Autodesk Inventor part; units mm, degrees
(part 2 of 3)
sketch "Sketch3" plane through (0, 0, 0) normal (0, 0, -1) x (-1, 0, 0)
  line L0 (-53.5235, -6.5875) -> (-53.5235, 0.9125)
  line L1 (5.4544, -6.5875) -> (-53.5235, -6.5875)
  line L2 (5.4544, 0.9125) -> (5.4544, -6.5875)
  line L3 (2.5944, 0.9125) -> (5.4544, 0.9125)
  arc A0 (2.5944, 0.9125) -> (2.4065, 0.7809) centre (2.5944, 0.7125) ccw
  line L4 (2.2868, 0.452) -> (2.4065, 0.7809)
  arc A1 (2.0617, 0.2877) -> (2.2868, 0.452) centre (2.0518, 0.5375) ccw
  arc A2 (2.0617, 0.2877) -> (2.0715, 0.2875) centre (2.0715, 0.5375) ccw
  line L5 (2.0518, 0.2875) -> (2.0715, 0.2875)
  arc A3 (2.0518, 0.2875) -> (2.0617, 0.2877) centre (2.0518, 0.5375) ccw
  arc A4 (1.8366, 0.452) -> (2.0617, 0.2877) centre (2.0715, 0.5375) ccw
  line L6 (1.5109, 1.3467) -> (1.8366, 0.452)
  arc A5 (1.5109, 1.3467) -> (1.417, 1.4125) centre (1.417, 1.3125) ccw
  line L7 (1.1356, 1.4125) -> (1.417, 1.4125)
  arc A6 (1.1356, 1.4125) -> (1.0416, 1.3467) centre (1.1356, 1.3125) ccw
  line L8 (0.716, 0.452) -> (1.0416, 1.3467)
  arc A7 (0.4909, 0.2877) -> (0.716, 0.452) centre (0.481, 0.5375) ccw
  arc A8 (0.4909, 0.2877) -> (0.5007, 0.2875) centre (0.5007, 0.5375) ccw
  line L9 (0.481, 0.2875) -> (0.5007, 0.2875)
  arc A9 (0.481, 0.2875) -> (0.4909, 0.2877) centre (0.481, 0.5375) ccw
  arc A10 (0.2658, 0.452) -> (0.4909, 0.2877) centre (0.5007, 0.5375) ccw
  line L10 (-0.0599, 1.3467) -> (0.2658, 0.452)
  arc A11 (-0.0599, 1.3467) -> (-0.1538, 1.4125) centre (-0.1538, 1.3125) ccw
  line L11 (-0.4352, 1.4125) -> (-0.1538, 1.4125)
  arc A12 (-0.4352, 1.4125) -> (-0.5292, 1.3467) centre (-0.4352, 1.3125) ccw
  line L12 (-0.8548, 0.452) -> (-0.5292, 1.3467)
  arc A13 (-1.0799, 0.2877) -> (-0.8548, 0.452) centre (-1.0898, 0.5375) ccw
  arc A14 (-1.0799, 0.2877) -> (-1.0701, 0.2875) centre (-1.0701, 0.5375) ccw
  line L13 (-1.0898, 0.2875) -> (-1.0701, 0.2875)
  arc A15 (-1.0898, 0.2875) -> (-1.0799, 0.2877) centre (-1.0898, 0.5375) ccw
  arc A16 (-1.305, 0.452) -> (-1.0799, 0.2877) centre (-1.0701, 0.5375) ccw
  line L14 (-1.6307, 1.3467) -> (-1.305, 0.452)
  arc A17 (-1.6307, 1.3467) -> (-1.7246, 1.4125) centre (-1.7246, 1.3125) ccw
  line L15 (-2.006, 1.4125) -> (-1.7246, 1.4125)
  arc A18 (-2.006, 1.4125) -> (-2.1, 1.3467) centre (-2.006, 1.3125) ccw
  line L16 (-2.4256, 0.452) -> (-2.1, 1.3467)
  arc A19 (-2.6507, 0.2877) -> (-2.4256, 0.452) centre (-2.6606, 0.5375) ccw
  arc A20 (-2.6507, 0.2877) -> (-2.6409, 0.2875) centre (-2.6409, 0.5375) ccw
  line L17 (-2.6606, 0.2875) -> (-2.6409, 0.2875)
  arc A21 (-2.6606, 0.2875) -> (-2.6507, 0.2877) centre (-2.6606, 0.5375) ccw
  arc A22 (-2.8758, 0.452) -> (-2.6507, 0.2877) centre (-2.6409, 0.5375) ccw
  line L18 (-3.2015, 1.3467) -> (-2.8758, 0.452)
  arc A23 (-3.2015, 1.3467) -> (-3.2954, 1.4125) centre (-3.2954, 1.3125) ccw
  line L19 (-3.5768, 1.4125) -> (-3.2954, 1.4125)
  arc A24 (-3.5768, 1.4125) -> (-3.6708, 1.3467) centre (-3.5768, 1.3125) ccw
  line L20 (-3.9964, 0.452) -> (-3.6708, 1.3467)
  arc A25 (-4.2215, 0.2877) -> (-3.9964, 0.452) centre (-4.2313, 0.5375) ccw
  arc A26 (-4.2215, 0.2877) -> (-4.2117, 0.2875) centre (-4.2117, 0.5375) ccw
  line L21 (-4.2313, 0.2875) -> (-4.2117, 0.2875)
  arc A27 (-4.2313, 0.2875) -> (-4.2215, 0.2877) centre (-4.2313, 0.5375) ccw
  arc A28 (-4.4466, 0.452) -> (-4.2215, 0.2877) centre (-4.2117, 0.5375) ccw
  line L22 (-4.7723, 1.3467) -> (-4.4466, 0.452)
  arc A29 (-4.7723, 1.3467) -> (-4.8662, 1.4125) centre (-4.8662, 1.3125) ccw
  line L23 (-5.1476, 1.4125) -> (-4.8662, 1.4125)
  arc A30 (-5.1476, 1.4125) -> (-5.2416, 1.3467) centre (-5.1476, 1.3125) ccw
  line L24 (-5.5672, 0.452) -> (-5.2416, 1.3467)
  arc A31 (-5.7923, 0.2877) -> (-5.5672, 0.452) centre (-5.8021, 0.5375) ccw
  arc A32 (-5.7923, 0.2877) -> (-5.7825, 0.2875) centre (-5.7825, 0.5375) ccw
  line L25 (-5.8021, 0.2875) -> (-5.7825, 0.2875)
  arc A33 (-5.8021, 0.2875) -> (-5.7923, 0.2877) centre (-5.8021, 0.5375) ccw
  arc A34 (-6.0174, 0.452) -> (-5.7923, 0.2877) centre (-5.7825, 0.5375) ccw
  line L26 (-6.343, 1.3467) -> (-6.0174, 0.452)
  arc A35 (-6.343, 1.3467) -> (-6.437, 1.4125) centre (-6.437, 1.3125) ccw
  line L27 (-6.7184, 1.4125) -> (-6.437, 1.4125)
  arc A36 (-6.7184, 1.4125) -> (-6.8124, 1.3467) centre (-6.7184, 1.3125) ccw
  line L28 (-7.138, 0.452) -> (-6.8124, 1.3467)
  arc A37 (-7.3631, 0.2877) -> (-7.138, 0.452) centre (-7.3729, 0.5375) ccw
  arc A38 (-7.3631, 0.2877) -> (-7.3533, 0.2875) centre (-7.3533, 0.5375) ccw
  line L29 (-7.3729, 0.2875) -> (-7.3533, 0.2875)
  arc A39 (-7.3729, 0.2875) -> (-7.3631, 0.2877) centre (-7.3729, 0.5375) ccw
  arc A40 (-7.5882, 0.452) -> (-7.3631, 0.2877) centre (-7.3533, 0.5375) ccw
  line L30 (-7.9138, 1.3467) -> (-7.5882, 0.452)
  arc A41 (-7.9138, 1.3467) -> (-8.0078, 1.4125) centre (-8.0078, 1.3125) ccw
  line L31 (-8.2892, 1.4125) -> (-8.0078, 1.4125)
  arc A42 (-8.2892, 1.4125) -> (-8.3832, 1.3467) centre (-8.2892, 1.3125) ccw
  line L32 (-8.7088, 0.452) -> (-8.3832, 1.3467)
  arc A43 (-8.9339, 0.2877) -> (-8.7088, 0.452) centre (-8.9437, 0.5375) ccw
  arc A44 (-8.9339, 0.2877) -> (-8.9241, 0.2875) centre (-8.9241, 0.5375) ccw
  line L33 (-8.9437, 0.2875) -> (-8.9241, 0.2875)
  arc A45 (-8.9437, 0.2875) -> (-8.9339, 0.2877) centre (-8.9437, 0.5375) ccw
  arc A46 (-9.159, 0.452) -> (-8.9339, 0.2877) centre (-8.9241, 0.5375) ccw
  line L34 (-9.4846, 1.3467) -> (-9.159, 0.452)
  arc A47 (-9.4846, 1.3467) -> (-9.5786, 1.4125) centre (-9.5786, 1.3125) ccw
  line L35 (-9.86, 1.4125) -> (-9.5786, 1.4125)
  arc A48 (-9.86, 1.4125) -> (-9.954, 1.3467) centre (-9.86, 1.3125) ccw
  line L36 (-10.2796, 0.452) -> (-9.954, 1.3467)
  arc A49 (-10.5047, 0.2877) -> (-10.2796, 0.452) centre (-10.5145, 0.5375) ccw
  arc A50 (-10.5047, 0.2877) -> (-10.4949, 0.2875) centre (-10.4949, 0.5375) ccw
  line L37 (-10.5145, 0.2875) -> (-10.4949, 0.2875)
  arc A51 (-10.5145, 0.2875) -> (-10.5047, 0.2877) centre (-10.5145, 0.5375) ccw
  arc A52 (-10.7298, 0.452) -> (-10.5047, 0.2877) centre (-10.4949, 0.5375) ccw
  line L38 (-11.0554, 1.3467) -> (-10.7298, 0.452)
  arc A53 (-11.0554, 1.3467) -> (-11.1494, 1.4125) centre (-11.1494, 1.3125) ccw
  line L39 (-11.4308, 1.4125) -> (-11.1494, 1.4125)
  arc A54 (-11.4308, 1.4125) -> (-11.5248, 1.3467) centre (-11.4308, 1.3125) ccw
  line L40 (-11.8504, 0.452) -> (-11.5248, 1.3467)
  arc A55 (-12.0755, 0.2877) -> (-11.8504, 0.452) centre (-12.0853, 0.5375) ccw
  arc A56 (-12.0755, 0.2877) -> (-12.0657, 0.2875) centre (-12.0657, 0.5375) ccw
  line L41 (-12.0853, 0.2875) -> (-12.0657, 0.2875)
  arc A57 (-12.0853, 0.2875) -> (-12.0755, 0.2877) centre (-12.0853, 0.5375) ccw
  arc A58 (-12.3006, 0.452) -> (-12.0755, 0.2877) centre (-12.0657, 0.5375) ccw
  line L42 (-12.6262, 1.3467) -> (-12.3006, 0.452)
  arc A59 (-12.6262, 1.3467) -> (-12.7202, 1.4125) centre (-12.7202, 1.3125) ccw
  line L43 (-13.0016, 1.4125) -> (-12.7202, 1.4125)
  arc A60 (-13.0016, 1.4125) -> (-13.0956, 1.3467) centre (-13.0016, 1.3125) ccw
  line L44 (-13.4212, 0.452) -> (-13.0956, 1.3467)
  arc A61 (-13.6463, 0.2877) -> (-13.4212, 0.452) centre (-13.6561, 0.5375) ccw
  arc A62 (-13.6463, 0.2877) -> (-13.6365, 0.2875) centre (-13.6365, 0.5375) ccw
  line L45 (-13.6561, 0.2875) -> (-13.6365, 0.2875)
  arc A63 (-13.6561, 0.2875) -> (-13.6463, 0.2877) centre (-13.6561, 0.5375) ccw
  arc A64 (-13.8714, 0.452) -> (-13.6463, 0.2877) centre (-13.6365, 0.5375) ccw
  line L46 (-14.197, 1.3467) -> (-13.8714, 0.452)
  arc A65 (-14.197, 1.3467) -> (-14.291, 1.4125) centre (-14.291, 1.3125) ccw
  line L47 (-14.5724, 1.4125) -> (-14.291, 1.4125)
  arc A66 (-14.5724, 1.4125) -> (-14.6664, 1.3467) centre (-14.5724, 1.3125) ccw
  line L48 (-14.992, 0.452) -> (-14.6664, 1.3467)
  arc A67 (-15.2171, 0.2877) -> (-14.992, 0.452) centre (-15.2269, 0.5375) ccw
  arc A68 (-15.2171, 0.2877) -> (-15.2073, 0.2875) centre (-15.2073, 0.5375) ccw
  line L49 (-15.2269, 0.2875) -> (-15.2073, 0.2875)
  arc A69 (-15.2269, 0.2875) -> (-15.2171, 0.2877) centre (-15.2269, 0.5375) ccw
  arc A70 (-15.4422, 0.452) -> (-15.2171, 0.2877) centre (-15.2073, 0.5375) ccw
  line L50 (-15.7678, 1.3467) -> (-15.4422, 0.452)
  arc A71 (-15.7678, 1.3467) -> (-15.8618, 1.4125) centre (-15.8618, 1.3125) ccw
  line L51 (-16.1432, 1.4125) -> (-15.8618, 1.4125)
  arc A72 (-16.1432, 1.4125) -> (-16.2372, 1.3467) centre (-16.1432, 1.3125) ccw
  line L52 (-16.5628, 0.452) -> (-16.2372, 1.3467)
  arc A73 (-16.7879, 0.2877) -> (-16.5628, 0.452) centre (-16.7977, 0.5375) ccw
  arc A74 (-16.7879, 0.2877) -> (-16.7781, 0.2875) centre (-16.7781, 0.5375) ccw
  line L53 (-16.7977, 0.2875) -> (-16.7781, 0.2875)
  arc A75 (-16.7977, 0.2875) -> (-16.7879, 0.2877) centre (-16.7977, 0.5375) ccw
  arc A76 (-17.013, 0.452) -> (-16.7879, 0.2877) centre (-16.7781, 0.5375) ccw
  line L54 (-17.3386, 1.3467) -> (-17.013, 0.452)
  arc A77 (-17.3386, 1.3467) -> (-17.4326, 1.4125) centre (-17.4326, 1.3125) ccw
  line L55 (-17.714, 1.4125) -> (-17.4326, 1.4125)
  arc A78 (-17.714, 1.4125) -> (-17.8079, 1.3467) centre (-17.714, 1.3125) ccw
  line L56 (-18.1336, 0.452) -> (-17.8079, 1.3467)
  arc A79 (-18.3587, 0.2877) -> (-18.1336, 0.452) centre (-18.3685, 0.5375) ccw
  arc A80 (-18.3587, 0.2877) -> (-18.3488, 0.2875) centre (-18.3488, 0.5375) ccw
  line L57 (-18.3685, 0.2875) -> (-18.3488, 0.2875)
  arc A81 (-18.3685, 0.2875) -> (-18.3587, 0.2877) centre (-18.3685, 0.5375) ccw
  arc A82 (-18.5838, 0.452) -> (-18.3587, 0.2877) centre (-18.3488, 0.5375) ccw
  line L58 (-18.9094, 1.3467) -> (-18.5838, 0.452)
  arc A83 (-18.9094, 1.3467) -> (-19.0034, 1.4125) centre (-19.0034, 1.3125) ccw
  line L59 (-19.2848, 1.4125) -> (-19.0034, 1.4125)
  arc A84 (-19.2848, 1.4125) -> (-19.3787, 1.3467) centre (-19.2848, 1.3125) ccw
  line L60 (-19.7044, 0.452) -> (-19.3787, 1.3467)
  arc A85 (-19.9295, 0.2877) -> (-19.7044, 0.452) centre (-19.9393, 0.5375) ccw
  arc A86 (-19.9295, 0.2877) -> (-19.9196, 0.2875) centre (-19.9196, 0.5375) ccw
  line L61 (-19.9393, 0.2875) -> (-19.9196, 0.2875)
  arc A87 (-19.9393, 0.2875) -> (-19.9295, 0.2877) centre (-19.9393, 0.5375) ccw
  arc A88 (-20.1546, 0.452) -> (-19.9295, 0.2877) centre (-19.9196, 0.5375) ccw
  line L62 (-20.4802, 1.3467) -> (-20.1546, 0.452)
  arc A89 (-20.4802, 1.3467) -> (-20.5742, 1.4125) centre (-20.5742, 1.3125) ccw
  line L63 (-20.8556, 1.4125) -> (-20.5742, 1.4125)
  arc A90 (-20.8556, 1.4125) -> (-20.9495, 1.3467) centre (-20.8556, 1.3125) ccw
  line L64 (-21.2752, 0.452) -> (-20.9495, 1.3467)
  arc A91 (-21.5003, 0.2877) -> (-21.2752, 0.452) centre (-21.5101, 0.5375) ccw
  arc A92 (-21.5003, 0.2877) -> (-21.4904, 0.2875) centre (-21.4904, 0.5375) ccw
  line L65 (-21.5101, 0.2875) -> (-21.4904, 0.2875)
  arc A93 (-21.5101, 0.2875) -> (-21.5003, 0.2877) centre (-21.5101, 0.5375) ccw
  arc A94 (-21.7254, 0.452) -> (-21.5003, 0.2877) centre (-21.4904, 0.5375) ccw
  line L66 (-22.051, 1.3467) -> (-21.7254, 0.452)
  arc A95 (-22.051, 1.3467) -> (-22.145, 1.4125) centre (-22.145, 1.3125) ccw
  line L67 (-22.4264, 1.4125) -> (-22.145, 1.4125)
  arc A96 (-22.4264, 1.4125) -> (-22.5203, 1.3467) centre (-22.4264, 1.3125) ccw
  line L68 (-22.846, 0.452) -> (-22.5203, 1.3467)
  arc A97 (-23.0711, 0.2877) -> (-22.846, 0.452) centre (-23.0809, 0.5375) ccw
  arc A98 (-23.0711, 0.2877) -> (-23.0612, 0.2875) centre (-23.0612, 0.5375) ccw
  line L69 (-23.0809, 0.2875) -> (-23.0612, 0.2875)
  arc A99 (-23.0809, 0.2875) -> (-23.0711, 0.2877) centre (-23.0809, 0.5375) ccw
  arc A100 (-23.2962, 0.452) -> (-23.0711, 0.2877) centre (-23.0612, 0.5375) ccw
  line L70 (-23.6218, 1.3467) -> (-23.2962, 0.452)
  arc A101 (-23.6218, 1.3467) -> (-23.7158, 1.4125) centre (-23.7158, 1.3125) ccw
  line L71 (-23.9972, 1.4125) -> (-23.7158, 1.4125)
  arc A102 (-23.9972, 1.4125) -> (-24.0911, 1.3467) centre (-23.9972, 1.3125) ccw
  line L72 (-24.4168, 0.452) -> (-24.0911, 1.3467)
  arc A103 (-24.6419, 0.2877) -> (-24.4168, 0.452) centre (-24.6517, 0.5375) ccw
  arc A104 (-24.6419, 0.2877) -> (-24.632, 0.2875) centre (-24.632, 0.5375) ccw
  line L73 (-24.6517, 0.2875) -> (-24.632, 0.2875)
  arc A105 (-24.6517, 0.2875) -> (-24.6419, 0.2877) centre (-24.6517, 0.5375) ccw
  arc A106 (-24.867, 0.452) -> (-24.6419, 0.2877) centre (-24.632, 0.5375) ccw
  line L74 (-25.1926, 1.3467) -> (-24.867, 0.452)
  arc A107 (-25.1926, 1.3467) -> (-25.2866, 1.4125) centre (-25.2866, 1.3125) ccw
  line L75 (-25.568, 1.4125) -> (-25.2866, 1.4125)
  arc A108 (-25.568, 1.4125) -> (-25.6619, 1.3467) centre (-25.568, 1.3125) ccw
  line L76 (-25.9876, 0.452) -> (-25.6619, 1.3467)
  arc A109 (-26.2127, 0.2877) -> (-25.9876, 0.452) centre (-26.2225, 0.5375) ccw
  arc A110 (-26.2127, 0.2877) -> (-26.2028, 0.2875) centre (-26.2028, 0.5375) ccw
  line L77 (-26.2225, 0.2875) -> (-26.2028, 0.2875)
  arc A111 (-26.2225, 0.2875) -> (-26.2127, 0.2877) centre (-26.2225, 0.5375) ccw
  arc A112 (-26.4378, 0.452) -> (-26.2127, 0.2877) centre (-26.2028, 0.5375) ccw
  line L78 (-26.7634, 1.3467) -> (-26.4378, 0.452)
  arc A113 (-26.7634, 1.3467) -> (-26.8574, 1.4125) centre (-26.8574, 1.3125) ccw
  line L79 (-27.1388, 1.4125) -> (-26.8574, 1.4125)
  arc A114 (-27.1388, 1.4125) -> (-27.2327, 1.3467) centre (-27.1388, 1.3125) ccw
  line L80 (-27.5584, 0.452) -> (-27.2327, 1.3467)
  arc A115 (-27.7835, 0.2877) -> (-27.5584, 0.452) centre (-27.7933, 0.5375) ccw
  arc A116 (-27.7835, 0.2877) -> (-27.7736, 0.2875) centre (-27.7736, 0.5375) ccw
  line L81 (-27.7933, 0.2875) -> (-27.7736, 0.2875)
  arc A117 (-27.7933, 0.2875) -> (-27.7835, 0.2877) centre (-27.7933, 0.5375) ccw
  arc A118 (-28.0085, 0.452) -> (-27.7835, 0.2877) centre (-27.7736, 0.5375) ccw
  line L82 (-28.3342, 1.3467) -> (-28.0085, 0.452)
  arc A119 (-28.3342, 1.3467) -> (-28.4282, 1.4125) centre (-28.4282, 1.3125) ccw
  line L83 (-28.7096, 1.4125) -> (-28.4282, 1.4125)
  arc A120 (-28.7096, 1.4125) -> (-28.8035, 1.3467) centre (-28.7096, 1.3125) ccw
  line L84 (-29.1292, 0.452) -> (-28.8035, 1.3467)
  arc A121 (-29.3543, 0.2877) -> (-29.1292, 0.452) centre (-29.3641, 0.5375) ccw
  arc A122 (-29.3543, 0.2877) -> (-29.3444, 0.2875) centre (-29.3444, 0.5375) ccw
  line L85 (-29.3641, 0.2875) -> (-29.3444, 0.2875)
  arc A123 (-29.3641, 0.2875) -> (-29.3543, 0.2877) centre (-29.3641, 0.5375) ccw
  arc A124 (-29.5793, 0.452) -> (-29.3543, 0.2877) centre (-29.3444, 0.5375) ccw
  line L86 (-29.905, 1.3467) -> (-29.5793, 0.452)
  arc A125 (-29.905, 1.3467) -> (-29.999, 1.4125) centre (-29.999, 1.3125) ccw
  line L87 (-30.2803, 1.4125) -> (-29.999, 1.4125)
  arc A126 (-30.2803, 1.4125) -> (-30.3743, 1.3467) centre (-30.2803, 1.3125) ccw
  line L88 (-30.7, 0.452) -> (-30.3743, 1.3467)
  arc A127 (-30.9251, 0.2877) -> (-30.7, 0.452) centre (-30.9349, 0.5375) ccw
  arc A128 (-30.9251, 0.2877) -> (-30.9152, 0.2875) centre (-30.9152, 0.5375) ccw
  line L89 (-30.9349, 0.2875) -> (-30.9152, 0.2875)
  arc A129 (-30.9349, 0.2875) -> (-30.9251, 0.2877) centre (-30.9349, 0.5375) ccw
  arc A130 (-31.1501, 0.452) -> (-30.9251, 0.2877) centre (-30.9152, 0.5375) ccw
  line L90 (-31.4758, 1.3467) -> (-31.1501, 0.452)
  arc A131 (-31.4758, 1.3467) -> (-31.5698, 1.4125) centre (-31.5698, 1.3125) ccw
  line L91 (-31.8511, 1.4125) -> (-31.5698, 1.4125)
  arc A132 (-31.8511, 1.4125) -> (-31.9451, 1.3467) centre (-31.8511, 1.3125) ccw
  line L92 (-32.2708, 0.452) -> (-31.9451, 1.3467)
  arc A133 (-32.4958, 0.2877) -> (-32.2708, 0.452) centre (-32.5057, 0.5375) ccw
  arc A134 (-32.4958, 0.2877) -> (-32.486, 0.2875) centre (-32.486, 0.5375) ccw
  line L93 (-32.5057, 0.2875) -> (-32.486, 0.2875)
  arc A135 (-32.5057, 0.2875) -> (-32.4958, 0.2877) centre (-32.5057, 0.5375) ccw
  arc A136 (-32.7209, 0.452) -> (-32.4958, 0.2877) centre (-32.486, 0.5375) ccw
  line L94 (-33.0466, 1.3467) -> (-32.7209, 0.452)
  arc A137 (-33.0466, 1.3467) -> (-33.1406, 1.4125) centre (-33.1406, 1.3125) ccw
  line L95 (-33.4219, 1.4125) -> (-33.1406, 1.4125)
  arc A138 (-33.4219, 1.4125) -> (-33.5159, 1.3467) centre (-33.4219, 1.3125) ccw
  line L96 (-33.8416, 0.452) -> (-33.5159, 1.3467)
  arc A139 (-34.0666, 0.2877) -> (-33.8416, 0.452) centre (-34.0765, 0.5375) ccw
  arc A140 (-34.0666, 0.2877) -> (-34.0568, 0.2875) centre (-34.0568, 0.5375) ccw
  line L97 (-34.0765, 0.2875) -> (-34.0568, 0.2875)
  arc A141 (-34.0765, 0.2875) -> (-34.0666, 0.2877) centre (-34.0765, 0.5375) ccw
  arc A142 (-34.2917, 0.452) -> (-34.0666, 0.2877) centre (-34.0568, 0.5375) ccw
  line L98 (-34.6174, 1.3467) -> (-34.2917, 0.452)
  arc A143 (-34.6174, 1.3467) -> (-34.7114, 1.4125) centre (-34.7114, 1.3125) ccw
  line L99 (-34.9927, 1.4125) -> (-34.7114, 1.4125)
  arc A144 (-34.9927, 1.4125) -> (-35.0867, 1.3467) centre (-34.9927, 1.3125) ccw
  line L100 (-35.4124, 0.452) -> (-35.0867, 1.3467)
  arc A145 (-35.6374, 0.2877) -> (-35.4124, 0.452) centre (-35.6473, 0.5375) ccw
  arc A146 (-35.6374, 0.2877) -> (-35.6276, 0.2875) centre (-35.6276, 0.5375) ccw
  line L101 (-35.6473, 0.2875) -> (-35.6276, 0.2875)
  arc A147 (-35.6473, 0.2875) -> (-35.6374, 0.2877) centre (-35.6473, 0.5375) ccw
  arc A148 (-35.8625, 0.452) -> (-35.6374, 0.2877) centre (-35.6276, 0.5375) ccw
  line L102 (-36.1882, 1.3467) -> (-35.8625, 0.452)
  arc A149 (-36.1882, 1.3467) -> (-36.2821, 1.4125) centre (-36.2821, 1.3125) ccw
  line L103 (-36.5635, 1.4125) -> (-36.2821, 1.4125)
  arc A150 (-36.5635, 1.4125) -> (-36.6575, 1.3467) centre (-36.5635, 1.3125) ccw
  line L104 (-36.9831, 0.452) -> (-36.6575, 1.3467)
  arc A151 (-37.2082, 0.2877) -> (-36.9831, 0.452) centre (-37.2181, 0.5375) ccw
  arc A152 (-37.2082, 0.2877) -> (-37.1984, 0.2875) centre (-37.1984, 0.5375) ccw
  line L105 (-37.2181, 0.2875) -> (-37.1984, 0.2875)
  arc A153 (-37.2181, 0.2875) -> (-37.2082, 0.2877) centre (-37.2181, 0.5375) ccw
  arc A154 (-37.4333, 0.452) -> (-37.2082, 0.2877) centre (-37.1984, 0.5375) ccw
  line L106 (-37.759, 1.3467) -> (-37.4333, 0.452)
  arc A155 (-37.759, 1.3467) -> (-37.8529, 1.4125) centre (-37.8529, 1.3125) ccw
  line L107 (-38.1343, 1.4125) -> (-37.8529, 1.4125)
  arc A156 (-38.1343, 1.4125) -> (-38.2283, 1.3467) centre (-38.1343, 1.3125) ccw
  line L108 (-38.5539, 0.452) -> (-38.2283, 1.3467)
  arc A157 (-38.779, 0.2877) -> (-38.5539, 0.452) centre (-38.7889, 0.5375) ccw
  arc A158 (-38.779, 0.2877) -> (-38.7692, 0.2875) centre (-38.7692, 0.5375) ccw
  line L109 (-38.7889, 0.2875) -> (-38.7692, 0.2875)
  arc A159 (-38.7889, 0.2875) -> (-38.779, 0.2877) centre (-38.7889, 0.5375) ccw
  arc A160 (-39.0041, 0.452) -> (-38.779, 0.2877) centre (-38.7692, 0.5375) ccw
  line L110 (-39.3298, 1.3467) -> (-39.0041, 0.452)
  arc A161 (-39.3298, 1.3467) -> (-39.4237, 1.4125) centre (-39.4237, 1.3125) ccw
  line L111 (-39.7051, 1.4125) -> (-39.4237, 1.4125)
  arc A162 (-39.7051, 1.4125) -> (-39.7991, 1.3467) centre (-39.7051, 1.3125) ccw
  line L112 (-40.1247, 0.452) -> (-39.7991, 1.3467)
  arc A163 (-40.3498, 0.2877) -> (-40.1247, 0.452) centre (-40.3597, 0.5375) ccw
  arc A164 (-40.3498, 0.2877) -> (-40.34, 0.2875) centre (-40.34, 0.5375) ccw
  line L113 (-40.3597, 0.2875) -> (-40.34, 0.2875)
  arc A165 (-40.3597, 0.2875) -> (-40.3498, 0.2877) centre (-40.3597, 0.5375) ccw
  arc A166 (-40.5749, 0.452) -> (-40.3498, 0.2877) centre (-40.34, 0.5375) ccw
  line L114 (-40.9006, 1.3467) -> (-40.5749, 0.452)
  arc A167 (-40.9006, 1.3467) -> (-40.9945, 1.4125) centre (-40.9945, 1.3125) ccw
  line L115 (-41.2759, 1.4125) -> (-40.9945, 1.4125)
  arc A168 (-41.2759, 1.4125) -> (-41.3699, 1.3467) centre (-41.2759, 1.3125) ccw
  line L116 (-41.6955, 0.452) -> (-41.3699, 1.3467)
  arc A169 (-41.9206, 0.2877) -> (-41.6955, 0.452) centre (-41.9305, 0.5375) ccw
  arc A170 (-41.9206, 0.2877) -> (-41.9108, 0.2875) centre (-41.9108, 0.5375) ccw
  line L117 (-41.9305, 0.2875) -> (-41.9108, 0.2875)
  arc A171 (-41.9305, 0.2875) -> (-41.9206, 0.2877) centre (-41.9305, 0.5375) ccw
  arc A172 (-42.1457, 0.452) -> (-41.9206, 0.2877) centre (-41.9108, 0.5375) ccw
  line L118 (-42.4714, 1.3467) -> (-42.1457, 0.452)
  arc A173 (-42.4714, 1.3467) -> (-42.5653, 1.4125) centre (-42.5653, 1.3125) ccw
  line L119 (-42.8467, 1.4125) -> (-42.5653, 1.4125)
  arc A174 (-42.8467, 1.4125) -> (-42.9407, 1.3467) centre (-42.8467, 1.3125) ccw
  line L120 (-43.2663, 0.452) -> (-42.9407, 1.3467)
  arc A175 (-43.4914, 0.2877) -> (-43.2663, 0.452) centre (-43.5013, 0.5375) ccw
  arc A176 (-43.4914, 0.2877) -> (-43.4816, 0.2875) centre (-43.4816, 0.5375) ccw
  line L121 (-43.5013, 0.2875) -> (-43.4816, 0.2875)
  arc A177 (-43.5013, 0.2875) -> (-43.4914, 0.2877) centre (-43.5013, 0.5375) ccw
  arc A178 (-43.7165, 0.452) -> (-43.4914, 0.2877) centre (-43.4816, 0.5375) ccw
  line L122 (-44.0422, 1.3467) -> (-43.7165, 0.452)
  arc A179 (-44.0422, 1.3467) -> (-44.1361, 1.4125) centre (-44.1361, 1.3125) ccw
  line L123 (-44.4175, 1.4125) -> (-44.1361, 1.4125)
  arc A180 (-44.4175, 1.4125) -> (-44.5115, 1.3467) centre (-44.4175, 1.3125) ccw
  line L124 (-44.8371, 0.452) -> (-44.5115, 1.3467)
  arc A181 (-45.0622, 0.2877) -> (-44.8371, 0.452) centre (-45.0721, 0.5375) ccw
  arc A182 (-45.0622, 0.2877) -> (-45.0524, 0.2875) centre (-45.0524, 0.5375) ccw
  line L125 (-45.0721, 0.2875) -> (-45.0524, 0.2875)
  arc A183 (-45.0721, 0.2875) -> (-45.0622, 0.2877) centre (-45.0721, 0.5375) ccw
  arc A184 (-45.2873, 0.452) -> (-45.0622, 0.2877) centre (-45.0524, 0.5375) ccw
  line L126 (-45.613, 1.3467) -> (-45.2873, 0.452)
  arc A185 (-45.613, 1.3467) -> (-45.7069, 1.4125) centre (-45.7069, 1.3125) ccw
  line L127 (-45.9883, 1.4125) -> (-45.7069, 1.4125)
  arc A186 (-45.9883, 1.4125) -> (-46.0823, 1.3467) centre (-45.9883, 1.3125) ccw
  line L128 (-46.4079, 0.452) -> (-46.0823, 1.3467)
  arc A187 (-46.633, 0.2877) -> (-46.4079, 0.452) centre (-46.6429, 0.5375) ccw
  arc A188 (-46.633, 0.2877) -> (-46.6232, 0.2875) centre (-46.6232, 0.5375) ccw
  line L129 (-46.6429, 0.2875) -> (-46.6232, 0.2875)
  arc A189 (-46.6429, 0.2875) -> (-46.633, 0.2877) centre (-46.6429, 0.5375) ccw
  arc A190 (-46.8581, 0.452) -> (-46.633, 0.2877) centre (-46.6232, 0.5375) ccw
  line L130 (-47.1838, 1.3467) -> (-46.8581, 0.452)
  arc A191 (-47.1838, 1.3467) -> (-47.2777, 1.4125) centre (-47.2777, 1.3125) ccw
  line L131 (-47.5591, 1.4125) -> (-47.2777, 1.4125)
  arc A192 (-47.5591, 1.4125) -> (-47.6531, 1.3467) centre (-47.5591, 1.3125) ccw
  line L132 (-47.9787, 0.452) -> (-47.6531, 1.3467)
  arc A193 (-48.2038, 0.2877) -> (-47.9787, 0.452) centre (-48.2136, 0.5375) ccw
  arc A194 (-48.2038, 0.2877) -> (-48.194, 0.2875) centre (-48.194, 0.5375) ccw
  line L133 (-48.2136, 0.2875) -> (-48.194, 0.2875)
  arc A195 (-48.2136, 0.2875) -> (-48.2038, 0.2877) centre (-48.2136, 0.5375) ccw
  arc A196 (-48.4289, 0.452) -> (-48.2038, 0.2877) centre (-48.194, 0.5375) ccw
  line L134 (-48.7545, 1.3467) -> (-48.4289, 0.452)
  arc A197 (-48.7545, 1.3467) -> (-48.8485, 1.4125) centre (-48.8485, 1.3125) ccw
  line L135 (-49.1299, 1.4125) -> (-48.8485, 1.4125)
  arc A198 (-49.1299, 1.4125) -> (-49.2239, 1.3467) centre (-49.1299, 1.3125) ccw
  line L136 (-49.5495, 0.452) -> (-49.2239, 1.3467)
  arc A199 (-49.7746, 0.2877) -> (-49.5495, 0.452) centre (-49.7844, 0.5375) ccw
  arc A200 (-49.7746, 0.2877) -> (-49.7648, 0.2875) centre (-49.7648, 0.5375) ccw
  line L137 (-49.7844, 0.2875) -> (-49.7648, 0.2875)
  arc A201 (-49.7844, 0.2875) -> (-49.7746, 0.2877) centre (-49.7844, 0.5375) ccw
  arc A202 (-49.9997, 0.452) -> (-49.7746, 0.2877) centre (-49.7648, 0.5375) ccw
  line L138 (-50.3253, 1.3467) -> (-49.9997, 0.452)
  arc A203 (-50.3253, 1.3467) -> (-50.4193, 1.4125) centre (-50.4193, 1.3125) ccw
  line L139 (-50.7007, 1.4125) -> (-50.4193, 1.4125)
  arc A204 (-50.7007, 1.4125) -> (-50.7947, 1.3467) centre (-50.7007, 1.3125) ccw
  line L140 (-51.1203, 0.452) -> (-50.7947, 1.3467)
  arc A205 (-51.3454, 0.2877) -> (-51.1203, 0.452) centre (-51.3552, 0.5375) ccw
  arc A206 (-51.3454, 0.2877) -> (-51.3356, 0.2875) centre (-51.3356, 0.5375) ccw
  line L141 (-51.3552, 0.2875) -> (-51.3356, 0.2875)
  arc A207 (-51.3552, 0.2875) -> (-51.3454, 0.2877) centre (-51.3552, 0.5375) ccw
  arc A208 (-51.5705, 0.452) -> (-51.3454, 0.2877) centre (-51.3356, 0.5375) ccw
  line L142 (-51.8961, 1.3467) -> (-51.5705, 0.452)
  arc A209 (-51.8961, 1.3467) -> (-51.9901, 1.4125) centre (-51.9901, 1.3125) ccw
  line L143 (-52.2715, 1.4125) -> (-51.9901, 1.4125)
  arc A210 (-52.2715, 1.4125) -> (-52.3655, 1.3467) centre (-52.2715, 1.3125) ccw
  line L144 (-52.4756, 1.0441) -> (-52.3655, 1.3467)
  arc A211 (-52.6635, 0.9125) -> (-52.4756, 1.0441) centre (-52.6635, 1.1125) ccw
  line L145 (-53.5235, 0.9125) -> (-52.6635, 0.9125)
  line L146 (-50.5235, -2.3375) -> (2.4544, -2.3375) construction
  line L147 (-50.5235, -3.6875) -> (2.4544, -3.6875)
  line L148 (2.4544, -0.9875) -> (-50.5235, -0.9875)
  arc A212 (-50.5235, -0.9875) -> (-50.5235, -3.6875) centre (-50.5235, -2.3375) ccw
  arc A213 (2.4544, -3.6875) -> (2.4544, -0.9875) centre (2.4544, -2.3375) ccw
  line L149 (-52.6635, 3.4125) -> (3.9478, 3.4125) construction
  line L150 (-50.5235, -0.4875) -> (2.4544, -0.4875)
  arc A214 (2.4544, -4.1875) -> (2.4544, -0.4875) centre (2.4544, -2.3375) ccw
  line L151 (2.4544, -4.1875) -> (-50.5235, -4.1875)
  arc A215 (-50.5235, -0.4875) -> (-50.5235, -4.1875) centre (-50.5235, -2.3375) ccw
  point P0 (0, 0)
  point P1 (-24.0346, -2.3375)
  dimension "d48" = 2.7
  dimension "d49" = 3
  dimension "d50" = 3
  dimension "d53" = 10
  dimension "d54" = 11.5
  dimension "d55" = 0.5
  constraints: 14 end point, 8 point on circle, 4 centre point, 4 tangent, 2 horizontal, 2 parallel, 1 midpoint, 3 other
  measures "d48" diameter of A213
  measures "d49" distance from line of L0 L146.start
  measures "d50" distance from line of L2 L146.end
  measures "d53" distance between parallel lines of L149 L1
  measures "d54" diameter of point (-24.035, -2.337) L149
  measures "d55" distance between parallel lines of L148 L150
extrude "Extrusion3" cut sketch "Sketch3" against normal up to surface (5 mm away) contours A212 L148 A213 L147
extrude "Extrusion4" cut sketch "Sketch3" against normal blind 0.3 contours A212 L148 A213 L147 | L150 A214 L151 A215
sketch "Sketch4" plane through (62.5235, -6.5875, 0) normal (1, 0, 0) x (0, 0, -1)
  line L0 (0, 0) -> (0, 7.5)
  line L1 (0, 7.5) -> (-5, 7.5)
  line L2 (35, 20) -> (-5, 20)
  line L3 (0, 7.5) -> (0, 20)
  line L4 (0, 11.8) -> (-5, 11.8)
  line L5 (-5, 11.8) -> (-5, 20)
  line L6 (-5, 20) -> (0, 20)
  point P0 (0, 6.5875)
  dimension "d58" = 8.2
  constraints: 8 end point, 3 perpendicular, 2 point on line, 1 collinear
  measures "d58" distance of L4.end L2.end
extrude "Extrusion5" cut sketch "Sketch4" against normal blind 10
sketch "Sketch5" plane through (62.5235, 5.2125, 0) normal (0, 0, 1) x (1, 0, 0)
  line L0 (-8.312, 0) -> (-7, 8.1999)
  line L1 (-8.312, 0) -> (-7, 8.1999)
  line L2 (0, 0) -> (-8.312, 0)
  line L3 (0, 8.2) -> (0, 0)
  line L4 (-7, 8.2) -> (0, 8.2)
  line L5 (-7, 8.1999) -> (-7, 8.2)
  point P0 (-62.5235, -5.2125)
extrude "Extrusion6" cut sketch "Sketch5" against normal blind 0.2
sketch "Sketch6" plane through (0, 0, 5) normal (0, 0, 1) x (1, 0, 0)
  line L0 (62.5235, 5.2125) -> (54.2115, 5.2125)
  line L1 (53.5235, 0.9125) -> (54.2115, 5.2125)
  line L2 (53.5235, 0.9125) -> (52.6635, 0.9125)
  arc A0 (52.4756, 1.0441) -> (52.6635, 0.9125) centre (52.6635, 1.1125) ccw
  line L3 (52.4756, 1.0441) -> (52.3655, 1.3467)
  arc A1 (52.3655, 1.3467) -> (52.2715, 1.4125) centre (52.2715, 1.3125) ccw
  line L4 (52.2715, 1.4125) -> (51.9901, 1.4125)
  arc A2 (51.9901, 1.4125) -> (51.8961, 1.3467) centre (51.9901, 1.3125) ccw
  line L5 (51.8961, 1.3467) -> (51.5705, 0.452)
  arc A3 (51.3454, 0.2877) -> (51.5705, 0.452) centre (51.3356, 0.5375) ccw
  arc A4 (51.3454, 0.2877) -> (51.3552, 0.2875) centre (51.3552, 0.5375) ccw
  line L6 (51.3552, 0.2875) -> (51.3356, 0.2875)
  arc A5 (51.3356, 0.2875) -> (51.3454, 0.2877) centre (51.3356, 0.5375) ccw
  arc A6 (51.1203, 0.452) -> (51.3454, 0.2877) centre (51.3552, 0.5375) ccw
  line L7 (51.1203, 0.452) -> (50.7947, 1.3467)
  arc A7 (50.7947, 1.3467) -> (50.7007, 1.4125) centre (50.7007, 1.3125) ccw
  line L8 (50.7007, 1.4125) -> (50.4193, 1.4125)
  arc A8 (50.4193, 1.4125) -> (50.3253, 1.3467) centre (50.4193, 1.3125) ccw
  line L9 (50.3253, 1.3467) -> (49.9997, 0.452)
  arc A9 (49.7746, 0.2877) -> (49.9997, 0.452) centre (49.7648, 0.5375) ccw
  arc A10 (49.7746, 0.2877) -> (49.7844, 0.2875) centre (49.7844, 0.5375) ccw
  line L10 (49.7844, 0.2875) -> (49.7648, 0.2875)
  arc A11 (49.7648, 0.2875) -> (49.7746, 0.2877) centre (49.7648, 0.5375) ccw
  arc A12 (49.5495, 0.452) -> (49.7746, 0.2877) centre (49.7844, 0.5375) ccw
  line L11 (49.5495, 0.452) -> (49.2239, 1.3467)
  arc A13 (49.2239, 1.3467) -> (49.1299, 1.4125) centre (49.1299, 1.3125) ccw
  line L12 (49.1299, 1.4125) -> (48.8485, 1.4125)
  arc A14 (48.8485, 1.4125) -> (48.7545, 1.3467) centre (48.8485, 1.3125) ccw
  line L13 (48.7545, 1.3467) -> (48.4289, 0.452)
  arc A15 (48.2038, 0.2877) -> (48.4289, 0.452) centre (48.194, 0.5375) ccw
  arc A16 (48.2038, 0.2877) -> (48.2136, 0.2875) centre (48.2136, 0.5375) ccw
  line L14 (48.2136, 0.2875) -> (48.194, 0.2875)
  arc A17 (48.194, 0.2875) -> (48.2038, 0.2877) centre (48.194, 0.5375) ccw
  arc A18 (47.9787, 0.452) -> (48.2038, 0.2877) centre (48.2136, 0.5375) ccw
  line L15 (47.9787, 0.452) -> (47.6531, 1.3467)
  arc A19 (47.6531, 1.3467) -> (47.5591, 1.4125) centre (47.5591, 1.3125) ccw
  line L16 (47.5591, 1.4125) -> (47.2777, 1.4125)
  arc A20 (47.2777, 1.4125) -> (47.1838, 1.3467) centre (47.2777, 1.3125) ccw
  line L17 (47.1838, 1.3467) -> (46.8581, 0.452)
  arc A21 (46.633, 0.2877) -> (46.8581, 0.452) centre (46.6232, 0.5375) ccw
  arc A22 (46.633, 0.2877) -> (46.6429, 0.2875) centre (46.6429, 0.5375) ccw
  line L18 (46.6429, 0.2875) -> (46.6232, 0.2875)
  arc A23 (46.6232, 0.2875) -> (46.633, 0.2877) centre (46.6232, 0.5375) ccw
  arc A24 (46.4079, 0.452) -> (46.633, 0.2877) centre (46.6429, 0.5375) ccw
  line L19 (46.4079, 0.452) -> (46.0823, 1.3467)
  arc A25 (46.0823, 1.3467) -> (45.9883, 1.4125) centre (45.9883, 1.3125) ccw
  line L20 (45.9883, 1.4125) -> (45.7069, 1.4125)
  arc A26 (45.7069, 1.4125) -> (45.613, 1.3467) centre (45.7069, 1.3125) ccw
  line L21 (45.613, 1.3467) -> (45.2873, 0.452)
  arc A27 (45.0622, 0.2877) -> (45.2873, 0.452) centre (45.0524, 0.5375) ccw
  arc A28 (45.0622, 0.2877) -> (45.0721, 0.2875) centre (45.0721, 0.5375) ccw
  line L22 (45.0721, 0.2875) -> (45.0524, 0.2875)
  arc A29 (45.0524, 0.2875) -> (45.0622, 0.2877) centre (45.0524, 0.5375) ccw
  arc A30 (44.8371, 0.452) -> (45.0622, 0.2877) centre (45.0721, 0.5375) ccw
  line L23 (44.8371, 0.452) -> (44.5115, 1.3467)
  arc A31 (44.5115, 1.3467) -> (44.4175, 1.4125) centre (44.4175, 1.3125) ccw
  line L24 (44.4175, 1.4125) -> (44.1361, 1.4125)
  arc A32 (44.1361, 1.4125) -> (44.0422, 1.3467) centre (44.1361, 1.3125) ccw
  line L25 (44.0422, 1.3467) -> (43.7165, 0.452)
  arc A33 (43.4914, 0.2877) -> (43.7165, 0.452) centre (43.4816, 0.5375) ccw
  arc A34 (43.4914, 0.2877) -> (43.5013, 0.2875) centre (43.5013, 0.5375) ccw
  line L26 (43.5013, 0.2875) -> (43.4816, 0.2875)
  arc A35 (43.4816, 0.2875) -> (43.4914, 0.2877) centre (43.4816, 0.5375) ccw
  arc A36 (43.2663, 0.452) -> (43.4914, 0.2877) centre (43.5013, 0.5375) ccw
  line L27 (43.2663, 0.452) -> (42.9407, 1.3467)
  arc A37 (42.9407, 1.3467) -> (42.8467, 1.4125) centre (42.8467, 1.3125) ccw
  line L28 (42.8467, 1.4125) -> (42.5653, 1.4125)
  arc A38 (42.5653, 1.4125) -> (42.4714, 1.3467) centre (42.5653, 1.3125) ccw
  line L29 (42.4714, 1.3467) -> (42.1457, 0.452)
  arc A39 (41.9206, 0.2877) -> (42.1457, 0.452) centre (41.9108, 0.5375) ccw
  arc A40 (41.9206, 0.2877) -> (41.9305, 0.2875) centre (41.9305, 0.5375) ccw
  line L30 (41.9305, 0.2875) -> (41.9108, 0.2875)
  arc A41 (41.9108, 0.2875) -> (41.9206, 0.2877) centre (41.9108, 0.5375) ccw
  arc A42 (41.6955, 0.452) -> (41.9206, 0.2877) centre (41.9305, 0.5375) ccw
  line L31 (41.6955, 0.452) -> (41.3699, 1.3467)
  arc A43 (41.3699, 1.3467) -> (41.2759, 1.4125) centre (41.2759, 1.3125) ccw
  line L32 (41.2759, 1.4125) -> (40.9945, 1.4125)
  arc A44 (40.9945, 1.4125) -> (40.9006, 1.3467) centre (40.9945, 1.3125) ccw
  line L33 (40.9006, 1.3467) -> (40.5749, 0.452)
  arc A45 (40.3498, 0.2877) -> (40.5749, 0.452) centre (40.34, 0.5375) ccw
  arc A46 (40.3498, 0.2877) -> (40.3597, 0.2875) centre (40.3597, 0.5375) ccw
  line L34 (40.3597, 0.2875) -> (40.34, 0.2875)
  arc A47 (40.34, 0.2875) -> (40.3498, 0.2877) centre (40.34, 0.5375) ccw
  arc A48 (40.1247, 0.452) -> (40.3498, 0.2877) centre (40.3597, 0.5375) ccw
  line L35 (40.1247, 0.452) -> (39.7991, 1.3467)
  arc A49 (39.7991, 1.3467) -> (39.7051, 1.4125) centre (39.7051, 1.3125) ccw
  line L36 (39.7051, 1.4125) -> (39.4237, 1.4125)
  arc A50 (39.4237, 1.4125) -> (39.3298, 1.3467) centre (39.4237, 1.3125) ccw
  line L37 (39.3298, 1.3467) -> (39.0041, 0.452)
  arc A51 (38.779, 0.2877) -> (39.0041, 0.452) centre (38.7692, 0.5375) ccw
  arc A52 (38.779, 0.2877) -> (38.7889, 0.2875) centre (38.7889, 0.5375) ccw
  line L38 (38.7889, 0.2875) -> (38.7692, 0.2875)
  arc A53 (38.7692, 0.2875) -> (38.779, 0.2877) centre (38.7692, 0.5375) ccw
  arc A54 (38.5539, 0.452) -> (38.779, 0.2877) centre (38.7889, 0.5375) ccw
  line L39 (38.5539, 0.452) -> (38.2283, 1.3467)
  arc A55 (38.2283, 1.3467) -> (38.1343, 1.4125) centre (38.1343, 1.3125) ccw
  line L40 (38.1343, 1.4125) -> (37.8529, 1.4125)
  arc A56 (37.8529, 1.4125) -> (37.759, 1.3467) centre (37.8529, 1.3125) ccw
  line L41 (37.759, 1.3467) -> (37.4333, 0.452)
  arc A57 (37.2082, 0.2877) -> (37.4333, 0.452) centre (37.1984, 0.5375) ccw
  arc A58 (37.2082, 0.2877) -> (37.2181, 0.2875) centre (37.2181, 0.5375) ccw
  line L42 (37.2181, 0.2875) -> (37.1984, 0.2875)
  arc A59 (37.1984, 0.2875) -> (37.2082, 0.2877) centre (37.1984, 0.5375) ccw
  arc A60 (36.9831, 0.452) -> (37.2082, 0.2877) centre (37.2181, 0.5375) ccw
  line L43 (36.9831, 0.452) -> (36.6575, 1.3467)
  arc A61 (36.6575, 1.3467) -> (36.5635, 1.4125) centre (36.5635, 1.3125) ccw
  line L44 (36.5635, 1.4125) -> (36.2821, 1.4125)
  arc A62 (36.2821, 1.4125) -> (36.1882, 1.3467) centre (36.2821, 1.3125) ccw
  line L45 (36.1882, 1.3467) -> (35.8625, 0.452)
  arc A63 (35.6374, 0.2877) -> (35.8625, 0.452) centre (35.6276, 0.5375) ccw
  arc A64 (35.6374, 0.2877) -> (35.6473, 0.2875) centre (35.6473, 0.5375) ccw
  line L46 (35.6473, 0.2875) -> (35.6276, 0.2875)
  arc A65 (35.6276, 0.2875) -> (35.6374, 0.2877) centre (35.6276, 0.5375) ccw
  arc A66 (35.4124, 0.452) -> (35.6374, 0.2877) centre (35.6473, 0.5375) ccw
  line L47 (35.4124, 0.452) -> (35.0867, 1.3467)
  arc A67 (35.0867, 1.3467) -> (34.9927, 1.4125) centre (34.9927, 1.3125) ccw
  line L48 (34.9927, 1.4125) -> (34.7114, 1.4125)
  arc A68 (34.7114, 1.4125) -> (34.6174, 1.3467) centre (34.7114, 1.3125) ccw
  line L49 (34.6174, 1.3467) -> (34.2917, 0.452)
  arc A69 (34.0666, 0.2877) -> (34.2917, 0.452) centre (34.0568, 0.5375) ccw
  arc A70 (34.0666, 0.2877) -> (34.0765, 0.2875) centre (34.0765, 0.5375) ccw
  line L50 (34.0765, 0.2875) -> (34.0568, 0.2875)
  arc A71 (34.0568, 0.2875) -> (34.0666, 0.2877) centre (34.0568, 0.5375) ccw
  arc A72 (33.8416, 0.452) -> (34.0666, 0.2877) centre (34.0765, 0.5375) ccw
  line L51 (33.8416, 0.452) -> (33.5159, 1.3467)
  arc A73 (33.5159, 1.3467) -> (33.4219, 1.4125) centre (33.4219, 1.3125) ccw
  line L52 (33.4219, 1.4125) -> (33.1406, 1.4125)
  arc A74 (33.1406, 1.4125) -> (33.0466, 1.3467) centre (33.1406, 1.3125) ccw
  line L53 (33.0466, 1.3467) -> (32.7209, 0.452)
  arc A75 (32.4958, 0.2877) -> (32.7209, 0.452) centre (32.486, 0.5375) ccw
  arc A76 (32.4958, 0.2877) -> (32.5057, 0.2875) centre (32.5057, 0.5375) ccw
  line L54 (32.5057, 0.2875) -> (32.486, 0.2875)
  arc A77 (32.486, 0.2875) -> (32.4958, 0.2877) centre (32.486, 0.5375) ccw
  arc A78 (32.2708, 0.452) -> (32.4958, 0.2877) centre (32.5057, 0.5375) ccw
  line L55 (32.2708, 0.452) -> (31.9451, 1.3467)
  arc A79 (31.9451, 1.3467) -> (31.8511, 1.4125) centre (31.8511, 1.3125) ccw
  line L56 (31.8511, 1.4125) -> (31.5698, 1.4125)
  arc A80 (31.5698, 1.4125) -> (31.4758, 1.3467) centre (31.5698, 1.3125) ccw
  line L57 (31.4758, 1.3467) -> (31.1501, 0.452)
  arc A81 (30.9251, 0.2877) -> (31.1501, 0.452) centre (30.9152, 0.5375) ccw
  arc A82 (30.9251, 0.2877) -> (30.9349, 0.2875) centre (30.9349, 0.5375) ccw
  line L58 (30.9349, 0.2875) -> (30.9152, 0.2875)
  arc A83 (30.9152, 0.2875) -> (30.9251, 0.2877) centre (30.9152, 0.5375) ccw
  arc A84 (30.7, 0.452) -> (30.9251, 0.2877) centre (30.9349, 0.5375) ccw
  line L59 (30.7, 0.452) -> (30.3743, 1.3467)
  arc A85 (30.3743, 1.3467) -> (30.2803, 1.4125) centre (30.2803, 1.3125) ccw
  line L60 (30.2803, 1.4125) -> (29.999, 1.4125)
  arc A86 (29.999, 1.4125) -> (29.905, 1.3467) centre (29.999, 1.3125) ccw
  line L61 (29.905, 1.3467) -> (29.5793, 0.452)
  arc A87 (29.3543, 0.2877) -> (29.5793, 0.452) centre (29.3444, 0.5375) ccw
  arc A88 (29.3543, 0.2877) -> (29.3641, 0.2875) centre (29.3641, 0.5375) ccw
  line L62 (29.3641, 0.2875) -> (29.3444, 0.2875)
  arc A89 (29.3444, 0.2875) -> (29.3543, 0.2877) centre (29.3444, 0.5375) ccw
  arc A90 (29.1292, 0.452) -> (29.3543, 0.2877) centre (29.3641, 0.5375) ccw
  line L63 (29.1292, 0.452) -> (28.8035, 1.3467)
  arc A91 (28.8035, 1.3467) -> (28.7096, 1.4125) centre (28.7096, 1.3125) ccw
  line L64 (28.7096, 1.4125) -> (28.4282, 1.4125)
  arc A92 (28.4282, 1.4125) -> (28.3342, 1.3467) centre (28.4282, 1.3125) ccw
  line L65 (28.3342, 1.3467) -> (28.0085, 0.452)
  arc A93 (27.7835, 0.2877) -> (28.0085, 0.452) centre (27.7736, 0.5375) ccw
  arc A94 (27.7835, 0.2877) -> (27.7933, 0.2875) centre (27.7933, 0.5375) ccw
  line L66 (27.7933, 0.2875) -> (27.7736, 0.2875)
  arc A95 (27.7736, 0.2875) -> (27.7835, 0.2877) centre (27.7736, 0.5375) ccw
  arc A96 (27.5584, 0.452) -> (27.7835, 0.2877) centre (27.7933, 0.5375) ccw
  line L67 (27.5584, 0.452) -> (27.2327, 1.3467)
  arc A97 (27.2327, 1.3467) -> (27.1388, 1.4125) centre (27.1388, 1.3125) ccw
  line L68 (27.1388, 1.4125) -> (26.8574, 1.4125)
  arc A98 (26.8574, 1.4125) -> (26.7634, 1.3467) centre (26.8574, 1.3125) ccw
  line L69 (26.7634, 1.3467) -> (26.4378, 0.452)
  arc A99 (26.2127, 0.2877) -> (26.4378, 0.452) centre (26.2028, 0.5375) ccw
  arc A100 (26.2127, 0.2877) -> (26.2225, 0.2875) centre (26.2225, 0.5375) ccw
  line L70 (26.2225, 0.2875) -> (26.2028, 0.2875)
  arc A101 (26.2028, 0.2875) -> (26.2127, 0.2877) centre (26.2028, 0.5375) ccw
  arc A102 (25.9876, 0.452) -> (26.2127, 0.2877) centre (26.2225, 0.5375) ccw
  line L71 (25.9876, 0.452) -> (25.6619, 1.3467)
  arc A103 (25.6619, 1.3467) -> (25.568, 1.4125) centre (25.568, 1.3125) ccw
  line L72 (25.568, 1.4125) -> (25.2866, 1.4125)
  arc A104 (25.2866, 1.4125) -> (25.1926, 1.3467) centre (25.2866, 1.3125) ccw
  line L73 (25.1926, 1.3467) -> (24.867, 0.452)
  arc A105 (24.6419, 0.2877) -> (24.867, 0.452) centre (24.632, 0.5375) ccw
  arc A106 (24.6419, 0.2877) -> (24.6517, 0.2875) centre (24.6517, 0.5375) ccw
  line L74 (24.6517, 0.2875) -> (24.632, 0.2875)
  arc A107 (24.632, 0.2875) -> (24.6419, 0.2877) centre (24.632, 0.5375) ccw
  arc A108 (24.4168, 0.452) -> (24.6419, 0.2877) centre (24.6517, 0.5375) ccw
  line L75 (24.4168, 0.452) -> (24.0911, 1.3467)
  arc A109 (24.0911, 1.3467) -> (23.9972, 1.4125) centre (23.9972, 1.3125) ccw
  line L76 (23.9972, 1.4125) -> (23.7158, 1.4125)
  arc A110 (23.7158, 1.4125) -> (23.6218, 1.3467) centre (23.7158, 1.3125) ccw
  line L77 (23.6218, 1.3467) -> (23.2962, 0.452)
  arc A111 (23.0711, 0.2877) -> (23.2962, 0.452) centre (23.0612, 0.5375) ccw
  arc A112 (23.0711, 0.2877) -> (23.0809, 0.2875) centre (23.0809, 0.5375) ccw
  line L78 (23.0809, 0.2875) -> (23.0612, 0.2875)
  arc A113 (23.0612, 0.2875) -> (23.0711, 0.2877) centre (23.0612, 0.5375) ccw
  arc A114 (22.846, 0.452) -> (23.0711, 0.2877) centre (23.0809, 0.5375) ccw
  line L79 (22.846, 0.452) -> (22.5203, 1.3467)
  arc A115 (22.5203, 1.3467) -> (22.4264, 1.4125) centre (22.4264, 1.3125) ccw
  line L80 (22.4264, 1.4125) -> (22.145, 1.4125)
  arc A116 (22.145, 1.4125) -> (22.051, 1.3467) centre (22.145, 1.3125) ccw
  line L81 (22.051, 1.3467) -> (21.7254, 0.452)
  arc A117 (21.5003, 0.2877) -> (21.7254, 0.452) centre (21.4904, 0.5375) ccw
  arc A118 (21.5003, 0.2877) -> (21.5101, 0.2875) centre (21.5101, 0.5375) ccw
  line L82 (21.5101, 0.2875) -> (21.4904, 0.2875)
  arc A119 (21.4904, 0.2875) -> (21.5003, 0.2877) centre (21.4904, 0.5375) ccw
  arc A120 (21.2752, 0.452) -> (21.5003, 0.2877) centre (21.5101, 0.5375) ccw
  line L83 (21.2752, 0.452) -> (20.9495, 1.3467)
  arc A121 (20.9495, 1.3467) -> (20.8556, 1.4125) centre (20.8556, 1.3125) ccw
  line L84 (20.8556, 1.4125) -> (20.5742, 1.4125)
  arc A122 (20.5742, 1.4125) -> (20.4802, 1.3467) centre (20.5742, 1.3125) ccw
  line L85 (20.4802, 1.3467) -> (20.1546, 0.452)
  arc A123 (19.9295, 0.2877) -> (20.1546, 0.452) centre (19.9196, 0.5375) ccw
  arc A124 (19.9295, 0.2877) -> (19.9393, 0.2875) centre (19.9393, 0.5375) ccw
  line L86 (19.9393, 0.2875) -> (19.9196, 0.2875)
  arc A125 (19.9196, 0.2875) -> (19.9295, 0.2877) centre (19.9196, 0.5375) ccw
  arc A126 (19.7044, 0.452) -> (19.9295, 0.2877) centre (19.9393, 0.5375) ccw
  line L87 (19.7044, 0.452) -> (19.3787, 1.3467)
  arc A127 (19.3787, 1.3467) -> (19.2848, 1.4125) centre (19.2848, 1.3125) ccw
  line L88 (19.2848, 1.4125) -> (19.0034, 1.4125)
  arc A128 (19.0034, 1.4125) -> (18.9094, 1.3467) centre (19.0034, 1.3125) ccw
  line L89 (18.9094, 1.3467) -> (18.5838, 0.452)
  arc A129 (18.3587, 0.2877) -> (18.5838, 0.452) centre (18.3488, 0.5375) ccw
  arc A130 (18.3587, 0.2877) -> (18.3685, 0.2875) centre (18.3685, 0.5375) ccw
  line L90 (18.3685, 0.2875) -> (18.3488, 0.2875)
  arc A131 (18.3488, 0.2875) -> (18.3587, 0.2877) centre (18.3488, 0.5375) ccw
  arc A132 (18.1336, 0.452) -> (18.3587, 0.2877) centre (18.3685, 0.5375) ccw
  line L91 (18.1336, 0.452) -> (17.8079, 1.3467)
  arc A133 (17.8079, 1.3467) -> (17.714, 1.4125) centre (17.714, 1.3125) ccw
  line L92 (17.714, 1.4125) -> (17.4326, 1.4125)
  arc A134 (17.4326, 1.4125) -> (17.3386, 1.3467) centre (17.4326, 1.3125) ccw
  line L93 (17.3386, 1.3467) -> (17.013, 0.452)
  arc A135 (16.7879, 0.2877) -> (17.013, 0.452) centre (16.7781, 0.5375) ccw
  arc A136 (16.7879, 0.2877) -> (16.7977, 0.2875) centre (16.7977, 0.5375) ccw
  line L94 (16.7977, 0.2875) -> (16.7781, 0.2875)
  arc A137 (16.7781, 0.2875) -> (16.7879, 0.2877) centre (16.7781, 0.5375) ccw
  arc A138 (16.5628, 0.452) -> (16.7879, 0.2877) centre (16.7977, 0.5375) ccw
  line L95 (16.5628, 0.452) -> (16.2372, 1.3467)
  arc A139 (16.2372, 1.3467) -> (16.1432, 1.4125) centre (16.1432, 1.3125) ccw
  line L96 (16.1432, 1.4125) -> (15.8618, 1.4125)
  arc A140 (15.8618, 1.4125) -> (15.7678, 1.3467) centre (15.8618, 1.3125) ccw
  line L97 (15.7678, 1.3467) -> (15.4422, 0.452)
  arc A141 (15.2171, 0.2877) -> (15.4422, 0.452) centre (15.2073, 0.5375) ccw
  arc A142 (15.2171, 0.2877) -> (15.2269, 0.2875) centre (15.2269, 0.5375) ccw
  line L98 (15.2269, 0.2875) -> (15.2073, 0.2875)
  arc A143 (15.2073, 0.2875) -> (15.2171, 0.2877) centre (15.2073, 0.5375) ccw
  arc A144 (14.992, 0.452) -> (15.2171, 0.2877) centre (15.2269, 0.5375) ccw
  line L99 (14.992, 0.452) -> (14.6664, 1.3467)
  arc A145 (14.6664, 1.3467) -> (14.5724, 1.4125) centre (14.5724, 1.3125) ccw
  line L100 (14.5724, 1.4125) -> (14.291, 1.4125)
  arc A146 (14.291, 1.4125) -> (14.197, 1.3467) centre (14.291, 1.3125) ccw
  line L101 (14.197, 1.3467) -> (13.8714, 0.452)
  arc A147 (13.6463, 0.2877) -> (13.8714, 0.452) centre (13.6365, 0.5375) ccw
  arc A148 (13.6463, 0.2877) -> (13.6561, 0.2875) centre (13.6561, 0.5375) ccw
  line L102 (13.6561, 0.2875) -> (13.6365, 0.2875)
  arc A149 (13.6365, 0.2875) -> (13.6463, 0.2877) centre (13.6365, 0.5375) ccw
  arc A150 (13.4212, 0.452) -> (13.6463, 0.2877) centre (13.6561, 0.5375) ccw
  line L103 (13.4212, 0.452) -> (13.0956, 1.3467)
  arc A151 (13.0956, 1.3467) -> (13.0016, 1.4125) centre (13.0016, 1.3125) ccw
  line L104 (13.0016, 1.4125) -> (12.7202, 1.4125)
  arc A152 (12.7202, 1.4125) -> (12.6262, 1.3467) centre (12.7202, 1.3125) ccw
  line L105 (12.6262, 1.3467) -> (12.3006, 0.452)
  arc A153 (12.0755, 0.2877) -> (12.3006, 0.452) centre (12.0657, 0.5375) ccw
  arc A154 (12.0755, 0.2877) -> (12.0853, 0.2875) centre (12.0853, 0.5375) ccw
  line L106 (12.0853, 0.2875) -> (12.0657, 0.2875)
  arc A155 (12.0657, 0.2875) -> (12.0755, 0.2877) centre (12.0657, 0.5375) ccw
  arc A156 (11.8504, 0.452) -> (12.0755, 0.2877) centre (12.0853, 0.5375) ccw
  line L107 (11.8504, 0.452) -> (11.5248, 1.3467)
  arc A157 (11.5248, 1.3467) -> (11.4308, 1.4125) centre (11.4308, 1.3125) ccw
  line L108 (11.4308, 1.4125) -> (11.1494, 1.4125)
  arc A158 (11.1494, 1.4125) -> (11.0554, 1.3467) centre (11.1494, 1.3125) ccw
  line L109 (11.0554, 1.3467) -> (10.7298, 0.452)
  arc A159 (10.5047, 0.2877) -> (10.7298, 0.452) centre (10.4949, 0.5375) ccw
  arc A160 (10.5047, 0.2877) -> (10.5145, 0.2875) centre (10.5145, 0.5375) ccw
  line L110 (10.5145, 0.2875) -> (10.4949, 0.2875)
  arc A161 (10.4949, 0.2875) -> (10.5047, 0.2877) centre (10.4949, 0.5375) ccw
  arc A162 (10.2796, 0.452) -> (10.5047, 0.2877) centre (10.5145, 0.5375) ccw
  line L111 (10.2796, 0.452) -> (9.954, 1.3467)
  arc A163 (9.954, 1.3467) -> (9.86, 1.4125) centre (9.86, 1.3125) ccw
  line L112 (9.86, 1.4125) -> (9.5786, 1.4125)
  arc A164 (9.5786, 1.4125) -> (9.4846, 1.3467) centre (9.5786, 1.3125) ccw
  line L113 (9.4846, 1.3467) -> (9.159, 0.452)
  arc A165 (8.9339, 0.2877) -> (9.159, 0.452) centre (8.9241, 0.5375) ccw
  arc A166 (8.9339, 0.2877) -> (8.9437, 0.2875) centre (8.9437, 0.5375) ccw
  line L114 (8.9437, 0.2875) -> (8.9241, 0.2875)
  arc A167 (8.9241, 0.2875) -> (8.9339, 0.2877) centre (8.9241, 0.5375) ccw
  arc A168 (8.7088, 0.452) -> (8.9339, 0.2877) centre (8.9437, 0.5375) ccw
  line L115 (8.7088, 0.452) -> (8.3832, 1.3467)
  arc A169 (8.3832, 1.3467) -> (8.2892, 1.4125) centre (8.2892, 1.3125) ccw
  line L116 (8.2892, 1.4125) -> (8.0078, 1.4125)
  arc A170 (8.0078, 1.4125) -> (7.9138, 1.3467) centre (8.0078, 1.3125) ccw
  line L117 (7.9138, 1.3467) -> (7.5882, 0.452)
  arc A171 (7.3631, 0.2877) -> (7.5882, 0.452) centre (7.3533, 0.5375) ccw
  arc A172 (7.3631, 0.2877) -> (7.3729, 0.2875) centre (7.3729, 0.5375) ccw
  line L118 (7.3729, 0.2875) -> (7.3533, 0.2875)
  arc A173 (7.3533, 0.2875) -> (7.3631, 0.2877) centre (7.3533, 0.5375) ccw
  arc A174 (7.138, 0.452) -> (7.3631, 0.2877) centre (7.3729, 0.5375) ccw
  line L119 (7.138, 0.452) -> (6.8124, 1.3467)
  arc A175 (6.8124, 1.3467) -> (6.7184, 1.4125) centre (6.7184, 1.3125) ccw
  line L120 (6.7184, 1.4125) -> (6.437, 1.4125)
  arc A176 (6.437, 1.4125) -> (6.343, 1.3467) centre (6.437, 1.3125) ccw
  line L121 (6.343, 1.3467) -> (6.0174, 0.452)
  arc A177 (5.7923, 0.2877) -> (6.0174, 0.452) centre (5.7825, 0.5375) ccw
  arc A178 (5.7923, 0.2877) -> (5.8021, 0.2875) centre (5.8021, 0.5375) ccw
  line L122 (5.8021, 0.2875) -> (5.7825, 0.2875)
  arc A179 (5.7825, 0.2875) -> (5.7923, 0.2877) centre (5.7825, 0.5375) ccw
  arc A180 (5.5672, 0.452) -> (5.7923, 0.2877) centre (5.8021, 0.5375) ccw
  line L123 (5.5672, 0.452) -> (5.2416, 1.3467)
  arc A181 (5.2416, 1.3467) -> (5.1476, 1.4125) centre (5.1476, 1.3125) ccw
  line L124 (5.1476, 1.4125) -> (4.8662, 1.4125)
  arc A182 (4.8662, 1.4125) -> (4.7723, 1.3467) centre (4.8662, 1.3125) ccw
  line L125 (4.7723, 1.3467) -> (4.4466, 0.452)
  arc A183 (4.2215, 0.2877) -> (4.4466, 0.452) centre (4.2117, 0.5375) ccw
  arc A184 (4.2215, 0.2877) -> (4.2313, 0.2875) centre (4.2313, 0.5375) ccw
  line L126 (4.2313, 0.2875) -> (4.2117, 0.2875)
  arc A185 (4.2117, 0.2875) -> (4.2215, 0.2877) centre (4.2117, 0.5375) ccw
  arc A186 (3.9964, 0.452) -> (4.2215, 0.2877) centre (4.2313, 0.5375) ccw
  line L127 (3.9964, 0.452) -> (3.6708, 1.3467)
  arc A187 (3.6708, 1.3467) -> (3.5768, 1.4125) centre (3.5768, 1.3125) ccw
  line L128 (3.5768, 1.4125) -> (3.2954, 1.4125)
  arc A188 (3.2954, 1.4125) -> (3.2015, 1.3467) centre (3.2954, 1.3125) ccw
  line L129 (3.2015, 1.3467) -> (2.8758, 0.452)
  arc A189 (2.6507, 0.2877) -> (2.8758, 0.452) centre (2.6409, 0.5375) ccw
  arc A190 (2.6507, 0.2877) -> (2.6606, 0.2875) centre (2.6606, 0.5375) ccw
  line L130 (2.6606, 0.2875) -> (2.6409, 0.2875)
  arc A191 (2.6409, 0.2875) -> (2.6507, 0.2877) centre (2.6409, 0.5375) ccw
  arc A192 (2.4256, 0.452) -> (2.6507, 0.2877) centre (2.6606, 0.5375) ccw
  line L131 (2.4256, 0.452) -> (2.1, 1.3467)
  arc A193 (2.1, 1.3467) -> (2.006, 1.4125) centre (2.006, 1.3125) ccw
  line L132 (2.006, 1.4125) -> (1.7246, 1.4125)
  arc A194 (1.7246, 1.4125) -> (1.6307, 1.3467) centre (1.7246, 1.3125) ccw
  line L133 (1.6307, 1.3467) -> (1.305, 0.452)
  arc A195 (1.0799, 0.2877) -> (1.305, 0.452) centre (1.0701, 0.5375) ccw
  arc A196 (1.0799, 0.2877) -> (1.0898, 0.2875) centre (1.0898, 0.5375) ccw
  line L134 (1.0898, 0.2875) -> (1.0701, 0.2875)
  arc A197 (1.0701, 0.2875) -> (1.0799, 0.2877) centre (1.0701, 0.5375) ccw
  arc A198 (0.8548, 0.452) -> (1.0799, 0.2877) centre (1.0898, 0.5375) ccw
  line L135 (0.8548, 0.452) -> (0.5292, 1.3467)
  arc A199 (0.5292, 1.3467) -> (0.4352, 1.4125) centre (0.4352, 1.3125) ccw
  line L136 (0.4352, 1.4125) -> (0.1538, 1.4125)
  arc A200 (0.1538, 1.4125) -> (0.0599, 1.3467) centre (0.1538, 1.3125) ccw
  line L137 (0.0599, 1.3467) -> (-0.2658, 0.452)
  arc A201 (-0.4909, 0.2877) -> (-0.2658, 0.452) centre (-0.5007, 0.5375) ccw
  arc A202 (-0.4909, 0.2877) -> (-0.481, 0.2875) centre (-0.481, 0.5375) ccw
  line L138 (-0.481, 0.2875) -> (-0.5007, 0.2875)
  arc A203 (-0.5007, 0.2875) -> (-0.4909, 0.2877) centre (-0.5007, 0.5375) ccw
  arc A204 (-0.716, 0.452) -> (-0.4909, 0.2877) centre (-0.481, 0.5375) ccw
  line L139 (-0.716, 0.452) -> (-1.0416, 1.3467)
  arc A205 (-1.0416, 1.3467) -> (-1.1356, 1.4125) centre (-1.1356, 1.3125) ccw
  line L140 (-1.1356, 1.4125) -> (-1.417, 1.4125)
  arc A206 (-1.417, 1.4125) -> (-1.5109, 1.3467) centre (-1.417, 1.3125) ccw